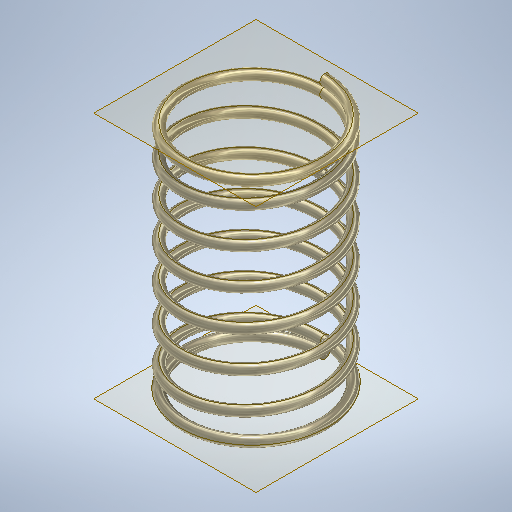
# Autodesk Inventor part: TR8_AntiBacklashNutCoil
Saved by Autodesk Inventor 2025.2 (Build 292293000, 293)
## iProperties
Created: 2017-03-01
Part Number: TR8_AntiBacklashNutCoil
Material: Ogólny
Document SubType Name: Modeling
Designer: user
Density: 1 g/cm^3
Appearance: Nickel
Author: user
Autodesk Inventor part; units mm, degrees
ref_plane "YZ Plane" through (0, 0, 0) normal (1, 0, 0) x (0, 1, 0)
ref_plane "XZ Plane" through (0, 0, 0) normal (0, 1, 0) x (-1, 0, 0)
sketch "Szkic1" plane through (0, 0, 0) normal (1, 0, 0) x (0, 1, 0)
  circle A0 centre (5.5, 0) radius 0.4
  line L0 (0, 0) -> (0, 2.2564)
  point P0 (0, 0)
  point P1 (0, 1.1282)
  dimension "d0" = 0.8
  dimension "d1" = 5.5
  constraints: 2 coincident, 2 end point, 1 centre point, 1 horizontal alignment, 1 midpoint, 1 vertical, 1 vertical alignment, 1 other
  measures "d0" diameter of A0
  measures "d1" distance from line of L0 point (5.5, 0)
coil "Zwój1" sketch "Szkic1" operation add axis through (0, 0, 0) along (0, 0, -1) pitch 0.9 turns 1 hand right
sketch "Szkic2" plane through (0, 5.5, 0) normal (-1, 0, 0) x (0, 0, 1)
  circle A0 centre (0, 0) radius 0.4 projected
  line L0 (0, -5.5) -> (2.2564, -5.5) projected
  point P0 (0, -5.5)
  point P1 (0, 0.4)
  constraints: 1 vertical alignment
coil "Zwój2" sketch "Szkic2" operation add axis through (0, 0, 0) along (0, 0, 1) pitch 2.8667 turns 6 hand right
sketch "Szkic3" plane through (0, 5.5, 17.2) normal (-1, 0, 0) x (0, 0, 1)
  circle A0 centre (0, 0) radius 0.4 projected
  line L0 (-17.2, -5.5) -> (-14.9436, -5.5) projected
  point P0 (-17.2, -5.5)
  point P1 (0.4, 0)
  constraints: 1 horizontal alignment
coil "Zwój3" sketch "Szkic3" operation add axis through (0, 0, 0) along (0, 0, 1) pitch 0.9 turns 1 hand right
sketch "Szkic4" plane through (0, 5.5, -0.9) normal (1, 0, 0) x (0, 0, -1)
  circle A0 centre (0, 0) radius 0.4 projected
  circle A1 centre (0, 0) radius 0.4 projected
  point P0 (-0.9, -5.5)
  point P1 (0, 0.4)
  point P2 (0.4, 0)
  constraints: 2 point on circle
ref_plane "Płaszczyzna konstrukcyjna1" through (0, 5.5, -1.3) normal (0, 0, 1) x (1, 0, 0)
sketch "Szkic5" plane through (0, 5.5, 18.1) normal (-1, 0, 0) x (0, 0, 1)
  circle A0 centre (0, 0) radius 0.4 projected
  point P0 (-18.1, -5.5)
  point P1 (0.4, 0)
  point P2 (0.4, 0)
  constraints: 1 coincident, 1 horizontal alignment
ref_plane "Płaszczyzna konstrukcyjna2" through (0, 5.5, 18.5) normal (0, 0, 1) x (1, 0, 0)
